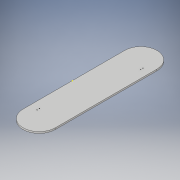
# Autodesk Inventor part: sfp_smartboard_upper_deck
Saved by Autodesk Inventor 2019 (Build 230136000, 136)
## iProperties
Created: 2019-02-09
Part Number: sfp_smartboard_upper_deck
Material: 一般
Document SubType Name: Modeling
Designer: drago
Density: 1 g/cm^3
Appearance: 既定
Author: drago
Autodesk Inventor part; units mm, degrees
ref_plane "YZ Plane" through (0, 0, 0) normal (1, 0, 0) x (0, 1, 0)
ref_plane "XZ Plane" through (0, 0, 0) normal (0, 1, 0) x (-1, 0, 0)
ref_plane "XY Plane" through (0, 0, 0) normal (0, 0, 1) x (1, 0, 0)
sketch "スケッチ1" plane through (0, 0, 0) normal (0, 1, 0) x (-1, 0, 0)
  point P0 (0, 0)
sketch "スケッチ2" plane through (0, 0, 0) normal (0, 1, 0) x (-1, 0, 0)
  line L0 (0.845, -60.969) -> (0.845, -330.969)
  line L1 (0, 0) -> (0, -1.5537)
  line L2 (-202.155, -60.969) -> (-202.155, -330.969)
  arc A0 (-202.155, -330.969) -> (0.845, -330.969) centre (-100.655, -330.969) ccw
  line L3 (0.845, -60.969) -> (0.845, 309.031)
  line L4 (-202.155, -60.969) -> (-202.155, 309.031)
  arc A1 (0.845, 309.031) -> (-202.155, 309.031) centre (-100.655, 309.031) ccw
  circle A2 centre (-47.655, 289.031) radius 6
  circle A3 centre (-47.655, 274.031) radius 6
  circle A4 centre (-153.655, -310.969) radius 6
  circle A5 centre (-153.655, -295.969) radius 6
  dimension "d0" = 270
  dimension "d1" = 203
  dimension "d38" = 12
  dimension "d39" = 20
  dimension "d40" = 12
  dimension "d41" = 15
  dimension "d42" = 48.5
  dimension "d43" = 48.5
  dimension "d44" = 12
  dimension "d45" = 12
  dimension "d46" = 20
  dimension "d47" = 15
  dimension "d48" = 48.5
  dimension "d49" = 48.5
  constraints: 10 end point, 6 centre point, 4 point on circle, 3 vertical, 2 tangent, 1 parallel
  measures "d0" distance of L0.start L0.end
  measures "d1" distance of L0.start L2.start
  measures "d38" diameter of A2
  measures "d39" vertical distance of A2.centre A1.centre
  measures "d40" diameter of A3
  measures "d41" distance of A2.centre A3.centre
  measures "d42" distance from line of L3 A2.centre
  measures "d43" distance from line of L3 A3.centre
  measures "d44" diameter of A4
  measures "d45" diameter of A5
  measures "d46" vertical distance of A4.centre A0.centre
  measures "d47" distance of A5.centre A4.centre
  measures "d48" distance from line of L2 A4.centre
  measures "d49" distance from line of L2 A5.centre
extrude "押し出し1" add sketch "スケッチ2" against normal blind 10 contours L0 A0 L2 L4 A1 L3 | A2 | A3 | A4 | A5
sketch "スケッチ6" plane through (0, 0, 0) normal (0, 1, 0) x (1, 0, 0)
  circle A0 centre (153.655, 290.969) radius 6
  circle A1 centre (153.655, 275.969) radius 6
  arc A2 (202.155, 330.969) -> (-0.845, 330.969) centre (100.655, 330.969) ccw projected
  line L0 (202.155, 330.969) -> (202.155, -309.031) projected
  point P0 (0, 0)
  dimension "d50" = 12
  dimension "d51" = 12
  dimension "d52" = 40
  dimension "d53" = 48.5
  dimension "d54" = 48.5
  dimension "d55" = 15
  constraints: 2 centre point
  measures "d50" diameter of A0
  measures "d51" diameter of A1
  measures "d52" vertical distance of A2.centre A0.centre
  measures "d53" distance from line of L0 A0.centre
  measures "d54" distance from line of L0 A1.centre
  measures "d55" distance of A1.centre A0.centre
hole "穴4" at (153.655, 0, -290.969) at (153.655, 0, -275.969) direction (0, -1, 0) diameter 4.917 end through all thread size "M6x1" class "6H" standard "ANSI Metric M Profile"
sketch "スケッチ7" plane through (0, 0, 0) normal (0, 1, 0) x (1, 0, 0)
  circle A0 centre (47.655, -269.031) radius 6
  circle A1 centre (47.655, -254.031) radius 6
  line L0 (-0.845, -309.031) -> (-0.845, 330.969) projected
  arc A2 (-0.845, -309.031) -> (202.155, -309.031) centre (100.655, -309.031) ccw projected
  point P0 (0, 0)
  dimension "d63" = 12
  dimension "d64" = 12
  dimension "d65" = 48.5
  dimension "d66" = 48.5
  dimension "d67" = 40
  dimension "d68" = 15
  constraints: 2 centre point
  measures "d63" diameter of A0
  measures "d64" diameter of A1
  measures "d65" distance from line of L0 A1.centre
  measures "d66" distance from line of L0 A0.centre
  measures "d67" vertical distance of A2.centre A0.centre
  measures "d68" distance of A0.centre A1.centre
hole "穴5" at (47.655, 0, 254.031) at (47.655, 0, 269.031) direction (0, -1, 0) diameter 4.917 end through all thread size "M6x1" class "6H" standard "ANSI Metric M Profile"
